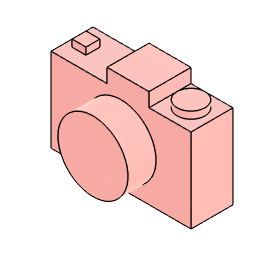
camera (1) (Autodesk Fusion 360 design; units mm, degrees)
part number: 2025-09-30-15-30-35-274
Autodesk Fusion 360 part; units mm, degrees
sketch "Sketch1" plane through (0, 0, 0) normal (0, 1, 0) x (1, 0, 0)
  line L0 (-50, -30) -> (50, -30)
  line L1 (50, -30) -> (50, 30)
  line L2 (50, 30) -> (-50, 30)
  line L3 (-50, 30) -> (-50, -30)
  dimension "d1" = 100
  dimension "d2" = 60
  constraint horizontal L0
  constraint vertical L1
  constraint horizontal L2
  constraint vertical L3
  measures "d1" distance of L0.start L0.end
  measures "d2" distance of L0.start L2.end
extrude "Extrude1" add sketch "Sketch1" along normal blind 30
sketch "Sketch2" plane through (0, 0, 0) normal (0, -1, 0) x (1, 0, 0)
  line L0 (-50, 30) -> (-50, -30)
  line L1 (-50, -30) -> (50, -30)
  line L2 (50, -30) -> (50, 30)
  line L3 (50, 30) -> (-50, 30)
  circle A0 centre (0, 0) radius 25
  dimension "d5" = 50
  constraint coincident A0.centre origin
  measures "d5" diameter of A0
extrude "Extrude2" add sketch "Sketch2" along normal blind 20 contours A0
sketch "Sketch3" plane through (0, 0, 30) normal (0, 0, 1) x (-1, 0, 0)
  line L0 (50, 0) -> (-50, 0)
  line L1 (-50, 0) -> (-50, -30)
  line L2 (-50, -30) -> (50, -30)
  line L3 (50, -30) -> (50, 0)
  circle A0 centre (-35, -15) radius 10
  dimension "d8" = 20
  dimension "d9" = 15
  measures "d8" diameter of A0
  measures "d9" distance of L1 A0.centre
extrude "Extrude3" add sketch "Sketch3" along normal blind 5 contours A0
sketch "Sketch4" plane through (0, 0, 30) normal (0, 0, 1) x (-1, 0, 0)
  circle A0 centre (-35, -15) radius 10
  line L0 (50, 0) -> (-50, 0)
  line L1 (-50, 0) -> (-50, -30)
  line L2 (-50, -30) -> (50, -30)
  line L3 (50, -30) -> (50, 0)
sketch "Sketch5" plane through (0, 0, 30) normal (0, 0, 1) x (-1, 0, 0)
  line L0 (-20, 0) -> (10, 0)
  line L1 (10, 0) -> (10, -30)
  line L2 (10, -30) -> (-20, -30)
  line L3 (-20, -30) -> (-20, 0)
  line L4 (-20, 0) -> (-10, -10)
  line L5 (10, 0) -> (25, 0)
  dimension "d12" = 30
  constraint horizontal L0
  constraint vertical L1
  constraint horizontal L2
  constraint vertical L3
  constraint perpendicular L1 L5
  measures "d12" distance of L1.end L2.end
extrude "Extrude4" add sketch "Sketch5" along normal blind 10
sketch "Sketch6" plane through (0, 0, 30) normal (0, 0, 1) x (-1, 0, 0)
  line L0 (-20, 0) -> (-10, -10)
  line L1 (35, -10) -> (45, -10)
  line L2 (45, -10) -> (45, -20)
  line L3 (45, -20) -> (35, -20)
  line L4 (35, -20) -> (35, -10)
  line L5 (35, -10) -> (45, -20) construction
  line L6 (45, -10) -> (35, -20) construction
  line L7 (50, -30) -> (50, 0)
  point P0 (40, -15)
  dimension "d15" = 15
  constraint horizontal L1
  constraint perpendicular L1 L2
  constraint parallel L1 L3
  constraint parallel L2 L4
  constraint coincident L5 P0
  constraint coincident L6 P0
  measures "d15" distance of L4 L7
extrude "Extrude5" add sketch "Sketch6" along normal blind 5
sketch "Sketch7" plane through (0, 0, 30) normal (0, 0, 1) x (-1, 0, 0)
